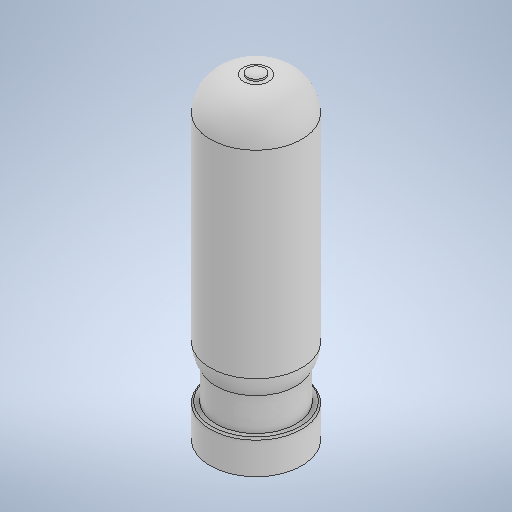
# Autodesk Inventor part: HY-H H2162–4T
Saved by Autodesk Inventor 2025 (Build 290162010, 162A)
## iProperties
Created: 2025-03-26
Part Number: HY-H H2162–4T
Material: Generic
Document SubType Name: Modeling
Designer: pokla
Density: 1 g/cm^3
Appearance: Default
Author: pokla
Autodesk Inventor part; units mm, degrees
ref_plane "YZ Plane" through (0, 0, 0) normal (1, 0, 0) x (0, 1, 0)
ref_plane "XZ Plane" through (0, 0, 0) normal (0, 1, 0) x (-1, 0, 0)
ref_plane "XY Plane" through (0, 0, 0) normal (0, 0, 1) x (1, 0, 0)
sketch "Sketch2" plane through (0, 0, 0) normal (0, 1, 0) x (-1, 0, 0)
  line L0 (0, 2130.997) -> (0, 0)
  line L1 (275, 1900) -> (75, 1900) construction
  line L2 (0, 1900) -> (0, 0)
  line L3 (0, 0) -> (275, 0)
  line L4 (275, 0) -> (275, 200)
  line L5 (275, 310) -> (75, 310) construction
  arc A0 (75, 310) -> (275, 510) centre (75, 510) ccw
  arc A1 (275, 1700) -> (75, 1900) centre (75, 1700) ccw
  line L6 (75, 1900) -> (0, 1900)
  line L7 (275, 1700) -> (275, 1900) construction
  line L8 (75, 310) -> (0, 310)
  line L9 (275, 310) -> (275, 510) construction
  line L10 (275, 510) -> (275, 1700)
  line L11 (275, 200) -> (240, 200)
  line L12 (240, 200) -> (240, 396.9735)
  line L13 (275, 200) -> (275, 310) construction
  line L14 (0, 1910) -> (50, 1910)
  line L15 (50, 1910) -> (50, 1900)
  point P0 (0, 1900)
  dimension "d3" = 550
  dimension "d7" = 200
  dimension "d8" = 200
  dimension "d9" = 35
  dimension "d10" = 200
  dimension "d12" = 50
  dimension "d13" = 10
  dimension "d14" = 1910
  dimension "d15" = 1600
  constraints: 32 end point, 8 parallel, 6 perpendicular, 5 point on circle, 5 tangent, 4 point on line, 3 horizontal, 2 centre point, 1 coincident, 1 vertical
  measures "d3" diameter of L4 L0
  measures "d7" radius of A1
  measures "d8" radius of A0
  measures "d9" distance of L4.end L11.end
  measures "d10" distance between parallel lines of L3 L11
  measures "d12" distance of L14.start L14.end
  measures "d13" distance between parallel lines of L6 L14
  measures "d14" distance between parallel lines of L3 L14
  measures "d15" distance between parallel lines of L5 L14
revolve "Revolution1" add sketch "Sketch2" angle 360 about axis through (0, 0, 2130.997) along (0, 0, -1)
chamfer "Chamfer1" distance 10 angle 45 1 edges at (275, 0, 200)
equation "\"d3\" = D"
equation "\"d8\" = d7"
equation "\"d14\" = H1"
equation "\"d15\" = H2"
equation "\"H1\" = 1910"
equation "\"H2\" = 1600"
equation "\"D\" = 550"
body "Solid1"
